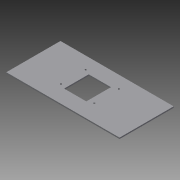
# Autodesk Inventor part: Winch baseplate
Saved by Autodesk Inventor 2015 SP1 (Build 190203100, 203)
## iProperties
Created: 2014-10-15
Part Number: Winch baseplate
Material: Generic
Document SubType Name: Modeling
Designer: aumccarville
Density: 1 g/cm^3
Appearance: Default
Author: aumccarville
Autodesk Inventor part; units mm, degrees
ref_plane "YZ Plane" through (0, 0, 0) normal (1, 0, 0) x (0, 1, 0)
ref_plane "XZ Plane" through (0, 0, 0) normal (0, 1, 0) x (-1, 0, 0)
ref_plane "XY Plane" through (0, 0, 0) normal (0, 0, 1) x (1, 0, 0)
sketch "Sketch1" plane through (0, 0, 0) normal (0, 0, 1) x (1, 0, 0)
  line L0 (0, 0) -> (292.1, 0)
  line L1 (292.1, 0) -> (292.1, 3.175)
  line L2 (292.1, 3.175) -> (0, 3.175)
  line L3 (0, 3.175) -> (0, 0)
  dimension "d0" = 292.1
  dimension "d1" = 3.175
  constraints: 8 end point, 2 parallel, 1 horizontal, 1 perpendicular
  measures "d0" distance of L2.end L1.end
  measures "d1" distance of L1.end L0.end
extrude "Extrusion1" add sketch "Sketch1" along normal blind 139.7
sketch "Sketch2" plane through (0, 3.175, 0) normal (0, 1, 0) x (1, 0, 0)
  point P0 (0, 0)
  point P1 (96.8502, -31.75)
  point P2 (96.8502, -95.25)
  point P3 (182.5498, -31.75)
  point P4 (182.5498, -95.25)
  dimension "d4" = 63.5
  dimension "d5" = 31.75
  dimension "d6" = 63.5
  dimension "d7" = 31.75
  dimension "d15" = 85.6996
  dimension "d16" = 85.6996
  dimension "d17" = 96.8502
  dimension "d18" = 96.8502
  measures "d4" distance of point (96.85, -95.25) point (96.85, -31.75)
  measures "d5" vertical distance of point (0, 0) point (96.85, -31.75)
  measures "d6" distance of point (182.55, -95.25) point (182.55, -31.75)
  measures "d7" vertical distance of point (0, 0) point (182.55, -31.75)
  measures "d15" distance of point (182.55, -31.75) point (96.85, -31.75)
  measures "d16" distance of point (96.85, -95.25) point (182.55, -95.25)
  measures "d17" horizontal distance of point (0, 0) point (96.85, -95.25)
  measures "d18" horizontal distance of point (0, 0) point (96.85, -31.75)
hole "Hole1" at (96.8502, 3.175, 31.75) at (96.8502, 3.175, 95.25) at (182.5498, 3.175, 31.75) at (182.5498, 3.175, 95.25) direction (0, -1, 0) diameter 4.1656 end through all
sketch "Sketch3" plane through (0, 3.175, 0) normal (0, 1, 0) x (1, 0, 0)
  line L0 (111.125, -38.1) -> (168.275, -38.1)
  line L1 (168.275, -38.1) -> (168.275, -101.6)
  line L2 (168.275, -101.6) -> (111.125, -101.6)
  line L3 (111.125, -101.6) -> (111.125, -38.1)
  line L4 (292.1, -139.7) -> (0, -139.7) projected
  point P0 (0, 0)
  dimension "d19" = 57.15
  dimension "d20" = 63.5
  dimension "d24" = 111.125
  dimension "d26" = 38.1
  constraints: 8 end point, 2 parallel, 1 horizontal, 1 perpendicular
  measures "d19" distance of L1.end L2.end
  measures "d20" distance between parallel lines of L2 L0
  measures "d24" distance from line of point (0, 0) L3
  measures "d26" vertical distance of L0.start point (0, 0)
extrude "Extrusion2" cut sketch "Sketch3" against normal blind 25.4
equation "\"d6\" = d4"
equation "\"d7\" = d5"
equation "\"d16\" = d15"
equation "\"d17\" = d18"
body "Solid1"
